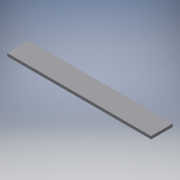
# Autodesk Inventor part: belt mockup
Saved by Autodesk Inventor 2016 (Build 200138000, 138)
## iProperties
Created: 2015-10-25
Part Number: belt mockup
Material: Rubber, Silicone
Document SubType Name: Modeling
Designer: as
Mass: 3.75 g
Surface Area: 34.6 cm^2
Volume: 3 cm^3
Density: 1.25 g/cm^3
Appearance: Rubber - Black
Author: as
Autodesk Inventor part; units mm, degrees
ref_plane "YZ Plane" through (0, 0, 0) normal (1, 0, 0) x (0, 1, 0)
ref_plane "XZ Plane" through (0, 0, 0) normal (0, 1, 0) x (-1, 0, 0)
ref_plane "XY Plane" through (0, 0, 0) normal (0, 0, 1) x (1, 0, 0)
sketch "Sketch1" plane through (0, 0, 0) normal (0, 0, 1) x (1, 0, 0)
  line L0 (-59.539, 0) -> (40.461, 0)
  line L1 (40.461, 0) -> (40.461, 15)
  line L2 (40.461, 15) -> (-59.539, 15)
  line L3 (-59.539, 15) -> (-59.539, 0)
  point P0 (0, 0)
  dimension "d0" = 100
  dimension "d1" = 15
  constraints: 8 end point, 2 parallel, 1 horizontal, 1 perpendicular
  measures "d0" distance of L0.start L0.end
  measures "d1" distance of L1.end L0.end
extrude "Extrusion1" add sketch "Sketch1" along normal blind 2
body "Solid1"
